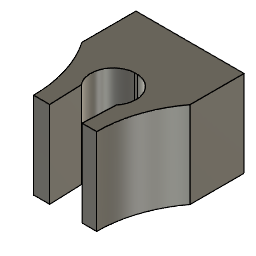
pieza (Autodesk Fusion 360 design; units mm, degrees)
Autodesk Fusion 360 part; units mm, degrees
sketch "Boceto1" plane through (0, 0, 0) normal (0, 1, 0) x (1, 0, 0)
  line L0 (-50, -60) -> (-40, -60)
  line L1 (-40, -60) -> (-40, -50)
  line L2 (-40, -50) -> (-50, -50)
  line L3 (-50, -50) -> (-50, -60)
  dimension "d1" = 10
  dimension "d2" = 10
  constraint horizontal L0
  constraint vertical L1
  constraint horizontal L2
  constraint vertical L3
  measures "d1" distance of L0.start L0.end
  measures "d2" distance of L0.start L2.end
extrude "Extruir1" add sketch "Boceto1" along normal blind 5
sketch "Boceto2" plane through (0, 0, 60) normal (0, 0, 1) x (-1, 0, 0)
  line L0 (50, 0) -> (40, 0)
  line L1 (40, 0) -> (40, -5)
  line L2 (40, -5) -> (50, -5)
  line L3 (50, -5) -> (50, 0)
  circle A0 centre (45, 2.0942) radius 2.1
  line L4 (48, 0) -> (42.1605, 0)
  line L5 (42.1605, 0) -> (42.1605, 6.4761)
  line L6 (42.1605, 6.4761) -> (48, 6.4761)
  line L7 (48, 6.4761) -> (48, 0)
  line L8 (46.6205, 3.4298) -> (43.3795, 3.4298)
  line L9 (45.0043, 6.4761) -> (43.5043, 6.4761)
  line L10 (45.0043, 6.4761) -> (46.5043, 6.4761)
  line L11 (46.6205, 3.4298) -> (46.5043, 6.4761)
  line L12 (43.3795, 3.4298) -> (43.5043, 6.4761)
  dimension "d5" = 4.2
  dimension "d6" = 1.5
  dimension "d7" = 1.5
  constraint horizontal L4
  constraint vertical L5
  constraint horizontal L6
  constraint vertical L7
  constraint coincident L0 L4.start
  constraint coincident A0 L8.start
  constraint coincident A0 L8.end
  constraint perpendicular L7 L8
  constraint coincident L6 L9.start
  constraint parallel L6 L9
  constraint parallel L6 L10
  measures "d5" diameter of A0
  measures "d6" distance of L9.start L9.end
  measures "d7" distance of L9.start L10.end
extrude "Extruir2" add sketch "Boceto2" against normal blind 10 contours L0 A0 L4 L6 L7 L11 | L0 A0 L4 L5 L6 L12
extrude "Extruir3" cut 1 faces at (-44.9481, 3.3333, 60) along direction (0, 0, -1) blind 2
fillet "Empalme1" radius 10.75 1 edges at (-42.1605, 0, 54)
fillet "Empalme2" radius 11.5 1 edges at (-48, 0, 54)
